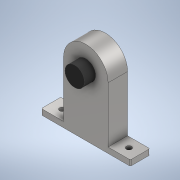
# Autodesk Inventor part: Stop sliding
Saved by Autodesk Inventor 2021 (Build 250183000, 183)
## iProperties
Created: 2021-06-07
Part Number: Stop sliding
Material: Generic
Document SubType Name: Modeling
Designer: Nelson
Density: 1 g/cm^3
Appearance: Default
Author: Nelson
Autodesk Inventor part; units mm, degrees
ref_plane "YZ Plane" through (0, 0, 0) normal (1, 0, 0) x (0, 1, 0)
ref_plane "XZ Plane" through (0, 0, 0) normal (0, 1, 0) x (-1, 0, 0)
ref_plane "XY Plane" through (0, 0, 0) normal (0, 0, 1) x (1, 0, 0)
sketch "Sketch3" plane through (0, 0, 0) normal (0, 0, 1) x (1, 0, 0)
  line L0 (0, 0) -> (80, 0)
  line L1 (80, 0) -> (80, 10)
  line L2 (80, 10) -> (40, 10)
  line L3 (40, 10) -> (40, 110)
  line L4 (0, 0) -> (0, 29.8306) construction
  line L5 (0, 0) -> (-80, 0)
  line L6 (-80, 0) -> (-80, 10)
  line L7 (-80, 10) -> (-40, 10)
  line L8 (-40, 10) -> (-40, 110)
  arc A0 (40, 110) -> (-40, 110) centre (0, 110) ccw
  dimension "d10" = 80
  dimension "d11" = 10
  dimension "d12" = 40
  dimension "d13" = 100
  dimension "d19" = 40
  constraints: 18 end point, 4 symmetric about line, 2 horizontal, 2 point on circle, 2 vertical, 1 centre point, 1 perpendicular
  measures "d10" distance of L0.start L0.end
  measures "d11" distance of L0.end L1.end
  measures "d12" distance of L1.end L2.end
  measures "d13" distance of L2.end L3.end
  measures "d19" radius of A0
extrude "Extrusion1" add sketch "Sketch3" against normal blind 35
sketch "Sketch4" plane through (0, 0, 0) normal (0, 0, 1) x (1, 0, 0)
  arc A0 (40, 110) -> (-40, 110) centre (0, 110) ccw projected
  circle A1 centre (0, 110) radius 17.5
  point P0 (0, 0)
  dimension "d20" = 35
  constraints: 1 centre point, 1 coincident
  measures "d20" diameter of A1
extrude "Extrusion2" add sketch "Sketch4" along normal blind 20
fillet "Fillet1" radius 2 4 edges at (80, 5, 0) (80, 5, -35) (-80, 5, 0) (-80, 5, -35)
sketch "Sketch5" plane through (-40, 10, 0) normal (0, 1, 0) x (1, 0, 0)
  line L0 (-38, 35) -> (0, 35) projected
  line L1 (80, 35) -> (118, 35) projected
  line L2 (-40, 2) -> (-40, 33) projected
  line L3 (120, 2) -> (120, 33) projected
  point P0 (40, 0)
  point P1 (-20, 17.5)
  point P2 (100, 17.5)
  dimension "d24" = 17.5
  dimension "d25" = 17.5
  dimension "d26" = 20
  dimension "d27" = 20
  measures "d24" distance from line of point (-20, 17.5) L0
  measures "d25" distance from line of L1 point (100, 17.5)
  measures "d26" distance from line of point (-20, 17.5) L2
  measures "d27" distance from line of point (100, 17.5) L3
hole "Hole1" at (-60, 10, -17.5) at (60, 10, -17.5) direction (0, -1, 0) diameter 9.5 depth 17.1 tip angle 137
equation "\"d25\" = d24"
equation "\"d27\" = d26"
body "Solid1"
